Autodesk Fusion 360 part; units mm, degrees
(part 2 of 8)
  spline S57 degree 5 poles (-37.4182, -68.8904) (-37.4192, -68.8954) (-37.4245, -68.9203) (-37.434, -68.9652) (-37.4475, -69.03) (-37.4649, -69.1149) (-37.4849, -69.2149) (-37.5045, -69.315) (-37.5237, -69.4153) (-37.5425, -69.5158) (-37.5608, -69.6164) (-37.5788, -69.7172) (-37.5963, -69.8182) (-37.6135, -69.9192) (-37.6302, -70.0204) (-37.6466, -70.1218) (-37.6626, -70.2233) (-37.6782, -70.3249) (-37.6934, -70.4267) (-37.7082, -70.5286) (-37.7227, -70.6307) (-37.7368, -70.7328) (-37.7505, -70.8351) (-37.7639, -70.9376) (-37.7769, -71.0401) (-37.7895, -71.1428) (-37.8018, -71.2456) (-37.8137, -71.3485) (-37.8253, -71.4515) (-37.8365, -71.5546) (-37.8474, -71.6579) (-37.8579, -71.7612) (-37.8681, -71.8647) (-37.878, -71.9683) (-37.8875, -72.072) (-37.8966, -72.1758) (-37.9054, -72.2797) (-37.9139, -72.3837) (-37.9221, -72.4878) (-37.9283, -72.5712) (-37.9329, -72.6338) (-37.9358, -72.6755) (-37.9373, -72.6964) knots 0.467834 0.467834 0.467834 0.467834 0.467834 0.467834 0.471429 0.485714 0.5 0.514286 0.528571 0.542857 0.557143 0.571429 0.585714 0.6 0.614286 0.628571 0.642857 0.657143 0.671429 0.685714 0.7 0.714286 0.728571 0.742857 0.757143 0.771429 0.785714 0.8 0.814286 0.828571 0.842857 0.857143 0.871429 0.885714 0.9 0.914286 0.928571 0.942857 0.957143 0.971429 0.985714 1 1 1 1 1 1
  arc A29 (-37.9373, -72.6964) -> (-36.5136, -73.4218) centre (0, 0) ccw
  spline S58 degree 5 poles (-36.5136, -73.4218) (-36.4976, -73.4083) (-36.4656, -73.3814) (-36.4176, -73.3409) (-36.3538, -73.2869) (-36.2744, -73.2191) (-36.1952, -73.1511) (-36.1164, -73.0829) (-36.0378, -73.0144) (-35.9595, -72.9458) (-35.8815, -72.877) (-35.8037, -72.8079) (-35.7263, -72.7386) (-35.6491, -72.6692) (-35.5723, -72.5995) (-35.4958, -72.5295) (-35.4195, -72.4594) (-35.3436, -72.389) (-35.2679, -72.3185) (-35.1926, -72.2477) (-35.1176, -72.1767) (-35.0429, -72.1054) (-34.9686, -72.034) (-34.8945, -71.9623) (-34.8208, -71.8904) (-34.7474, -71.8183) (-34.6743, -71.7459) (-34.6016, -71.6733) (-34.5292, -71.6005) (-34.4572, -71.5274) (-34.3855, -71.4541) (-34.3142, -71.3806) (-34.2432, -71.3069) (-34.1726, -71.2329) (-34.1023, -71.1586) (-34.0324, -71.0842) (-33.9629, -71.0094) (-33.8938, -70.9345) (-33.8353, -70.8705) (-33.7908, -70.8215) (-33.7601, -70.7874) (-33.7431, -70.7685) (-33.7396, -70.7647) knots -1 -1 -1 -1 -1 -1 -0.985714 -0.971429 -0.957143 -0.942857 -0.928571 -0.914286 -0.9 -0.885714 -0.871429 -0.857143 -0.842857 -0.828571 -0.814286 -0.8 -0.785714 -0.771429 -0.757143 -0.742857 -0.728571 -0.714286 -0.7 -0.685714 -0.671429 -0.657143 -0.642857 -0.628571 -0.614286 -0.6 -0.585714 -0.571429 -0.557143 -0.542857 -0.528571 -0.514286 -0.5 -0.485714 -0.471429 -0.467834 -0.467834 -0.467834 -0.467834 -0.467834 -0.467834
  spline S59 degree 3 poles (-32.5768, -70.5256) (-32.695, -70.471) (-32.8228, -70.44) (-33.083, -70.4288) (-33.2129, -70.4486) (-33.4127, -70.5206) (-33.4862, -70.5579) (-33.6225, -70.6496) (-33.6847, -70.7036) (-33.7396, -70.7647) knots 0 0 0 0 0.039064 0.039064 0.078129 0.078129 0.102767 0.102767 0.127404 0.127404 0.127404 0.127404
  arc A30 (-32.5768, -70.5256) -> (-32.4711, -70.5744) centre (0, 0) ccw
  spline S60 degree 3 poles (-31.8977, -71.6138) (-31.8807, -71.4847) (-31.889, -71.3535) (-31.9555, -71.1017) (-32.013, -70.9835) (-32.141, -70.8142) (-32.1984, -70.755) (-32.3264, -70.6521) (-32.3965, -70.6087) (-32.4711, -70.5744) knots 0 0 0 0 0.039064 0.039064 0.078129 0.078129 0.102767 0.102767 0.127404 0.127404 0.127404 0.127404
  spline S61 degree 5 poles (-31.8977, -71.6138) (-31.8984, -71.6189) (-31.9018, -71.6442) (-31.9077, -71.6896) (-31.9161, -71.7553) (-31.9267, -71.8413) (-31.9389, -71.9425) (-31.9505, -72.0439) (-31.9618, -72.1454) (-31.9726, -72.2471) (-31.983, -72.3488) (-31.993, -72.4507) (-32.0026, -72.5527) (-32.0117, -72.6548) (-32.0205, -72.757) (-32.0289, -72.8594) (-32.0368, -72.9618) (-32.0444, -73.0644) (-32.0516, -73.167) (-32.0584, -73.2698) (-32.0648, -73.3726) (-32.0708, -73.4756) (-32.0765, -73.5786) (-32.0818, -73.6818) (-32.0867, -73.785) (-32.0912, -73.8884) (-32.0954, -73.9918) (-32.0992, -74.0953) (-32.1027, -74.199) (-32.1058, -74.3027) (-32.1085, -74.4065) (-32.1109, -74.5103) (-32.1129, -74.6143) (-32.1146, -74.7183) (-32.116, -74.8224) (-32.1169, -74.9266) (-32.1176, -75.0309) (-32.1179, -75.1353) (-32.1178, -75.2397) (-32.1175, -75.3233) (-32.1172, -75.386) (-32.1168, -75.4279) (-32.1167, -75.4488) knots 0.467834 0.467834 0.467834 0.467834 0.467834 0.467834 0.471429 0.485714 0.5 0.514286 0.528571 0.542857 0.557143 0.571429 0.585714 0.6 0.614286 0.628571 0.642857 0.657143 0.671429 0.685714 0.7 0.714286 0.728571 0.742857 0.757143 0.771429 0.785714 0.8 0.814286 0.828571 0.842857 0.857143 0.871429 0.885714 0.9 0.914286 0.928571 0.942857 0.957143 0.971429 0.985714 1 1 1 1 1 1
  arc A31 (-32.1167, -75.4488) -> (-30.6404, -76.0603) centre (0, 0) ccw
  spline S62 degree 5 poles (-30.6404, -76.0603) (-30.6255, -76.0456) (-30.5957, -76.0162) (-30.5511, -75.9721) (-30.4917, -75.9132) (-30.4179, -75.8394) (-30.3443, -75.7654) (-30.271, -75.6912) (-30.198, -75.6169) (-30.1254, -75.5423) (-30.053, -75.4675) (-29.9809, -75.3926) (-29.9091, -75.3175) (-29.8377, -75.2421) (-29.7666, -75.1666) (-29.6957, -75.0909) (-29.6252, -75.015) (-29.555, -74.9389) (-29.4852, -74.8626) (-29.4156, -74.7861) (-29.3464, -74.7095) (-29.2776, -74.6326) (-29.209, -74.5555) (-29.1408, -74.4783) (-29.073, -74.4008) (-29.0055, -74.3231) (-28.9383, -74.2452) (-28.8715, -74.1672) (-28.8051, -74.0889) (-28.739, -74.0104) (-28.6733, -73.9317) (-28.6079, -73.8528) (-28.543, -73.7737) (-28.4784, -73.6944) (-28.4141, -73.6149) (-28.3503, -73.5352) (-28.2869, -73.4552) (-28.2238, -73.3751) (-28.1706, -73.3067) (-28.1301, -73.2543) (-28.1021, -73.218) (-28.0866, -73.1978) (-28.0835, -73.1937) knots -1 -1 -1 -1 -1 -1 -0.985714 -0.971429 -0.957143 -0.942857 -0.928571 -0.914286 -0.9 -0.885714 -0.871429 -0.857143 -0.842857 -0.828571 -0.814286 -0.8 -0.785714 -0.771429 -0.757143 -0.742857 -0.728571 -0.714286 -0.7 -0.685714 -0.671429 -0.657143 -0.642857 -0.628571 -0.614286 -0.6 -0.585714 -0.571429 -0.557143 -0.542857 -0.528571 -0.514286 -0.5 -0.485714 -0.471429 -0.467834 -0.467834 -0.467834 -0.467834 -0.467834 -0.467834
  spline S63 degree 3 poles (-26.943, -72.8642) (-27.0652, -72.819) (-27.195, -72.7981) (-27.4552, -72.8073) (-27.5832, -72.8373) (-27.7767, -72.9248) (-27.8471, -72.9677) (-27.9757, -73.0698) (-28.0335, -73.1286) (-28.0835, -73.1937) knots 0 0 0 0 0.039064 0.039064 0.078129 0.078129 0.102767 0.102767 0.127404 0.127404 0.127404 0.127404
  arc A32 (-26.943, -72.8642) -> (-26.8339, -72.9045) centre (0, 0) ccw
  spline S64 degree 3 poles (-26.1807, -73.8957) (-26.1738, -73.7657) (-26.1924, -73.6356) (-26.2784, -73.3897) (-26.345, -73.2764) (-26.4859, -73.1176) (-26.5478, -73.0631) (-26.6835, -72.9706) (-26.7568, -72.9328) (-26.8339, -72.9045) knots 0 0 0 0 0.039064 0.039064 0.078129 0.078129 0.102767 0.102767 0.127404 0.127404 0.127404 0.127404
  spline S65 degree 5 poles (-26.1807, -73.8957) (-26.1809, -73.9008) (-26.1823, -73.9263) (-26.1846, -73.9721) (-26.1878, -74.0382) (-26.1917, -74.1248) (-26.1959, -74.2267) (-26.1995, -74.3286) (-26.2028, -74.4307) (-26.2056, -74.5329) (-26.208, -74.6352) (-26.2099, -74.7375) (-26.2115, -74.8399) (-26.2126, -74.9424) (-26.2133, -75.045) (-26.2136, -75.1477) (-26.2136, -75.2505) (-26.2131, -75.3533) (-26.2122, -75.4562) (-26.2109, -75.5592) (-26.2092, -75.6622) (-26.2072, -75.7653) (-26.2047, -75.8685) (-26.2019, -75.9718) (-26.1987, -76.0751) (-26.1951, -76.1785) (-26.1912, -76.2819) (-26.1868, -76.3854) (-26.1821, -76.489) (-26.1771, -76.5926) (-26.1717, -76.6963) (-26.1659, -76.8) (-26.1598, -76.9038) (-26.1533, -77.0077) (-26.1464, -77.1116) (-26.1393, -77.2155) (-26.1317, -77.3195) (-26.1238, -77.4236) (-26.1156, -77.5277) (-26.1087, -77.611) (-26.1034, -77.6735) (-26.0998, -77.7152) (-26.098, -77.736) knots 0.467834 0.467834 0.467834 0.467834 0.467834 0.467834 0.471429 0.485714 0.5 0.514286 0.528571 0.542857 0.557143 0.571429 0.585714 0.6 0.614286 0.628571 0.642857 0.657143 0.671429 0.685714 0.7 0.714286 0.728571 0.742857 0.757143 0.771429 0.785714 0.8 0.814286 0.828571 0.842857 0.857143 0.871429 0.885714 0.9 0.914286 0.928571 0.942857 0.957143 0.971429 0.985714 1 1 1 1 1 1
  arc A33 (-26.098, -77.736) -> (-24.5784, -78.2298) centre (0, 0) ccw
  spline S66 degree 5 poles (-24.5784, -78.2298) (-24.5646, -78.214) (-24.5372, -78.1824) (-24.4962, -78.135) (-24.4417, -78.0716) (-24.3738, -77.9922) (-24.3063, -77.9127) (-24.239, -77.8329) (-24.1721, -77.7531) (-24.1055, -77.673) (-24.0392, -77.5928) (-23.9733, -77.5125) (-23.9076, -77.4319) (-23.8423, -77.3512) (-23.7773, -77.2704) (-23.7126, -77.1893) (-23.6483, -77.1081) (-23.5843, -77.0268) (-23.5206, -76.9452) (-23.4573, -76.8635) (-23.3943, -76.7817) (-23.3317, -76.6996) (-23.2694, -76.6174) (-23.2075, -76.535) (-23.1459, -76.4525) (-23.0847, -76.3697) (-23.0239, -76.2868) (-22.9634, -76.2038) (-22.9033, -76.1205) (-22.8436, -76.0371) (-22.7843, -75.9535) (-22.7253, -75.8697) (-22.6667, -75.7858) (-22.6086, -75.7016) (-22.5508, -75.6173) (-22.4934, -75.5328) (-22.4364, -75.4482) (-22.3799, -75.3633) (-22.3322, -75.291) (-22.2959, -75.2356) (-22.2709, -75.1972) (-22.257, -75.1758) (-22.2542, -75.1715) knots -1 -1 -1 -1 -1 -1 -0.985714 -0.971429 -0.957143 -0.942857 -0.928571 -0.914286 -0.9 -0.885714 -0.871429 -0.857143 -0.842857 -0.828571 -0.814286 -0.8 -0.785714 -0.771429 -0.757143 -0.742857 -0.728571 -0.714286 -0.7 -0.685714 -0.671429 -0.657143 -0.642857 -0.628571 -0.614286 -0.6 -0.585714 -0.571429 -0.557143 -0.542857 -0.528571 -0.514286 -0.5 -0.485714 -0.471429 -0.467834 -0.467834 -0.467834 -0.467834 -0.467834 -0.467834
  spline S67 degree 3 poles (-21.1431, -74.7535) (-21.2684, -74.718) (-21.3994, -74.7074) (-21.6582, -74.737) (-21.7834, -74.7769) (-21.9695, -74.8793) (-22.0363, -74.9276) (-22.1565, -75.0395) (-22.2095, -75.1026) (-22.2542, -75.1715) knots 0 0 0 0 0.039064 0.039064 0.078129 0.078129 0.102767 0.102767 0.127404 0.127404 0.127404 0.127404
  arc A34 (-21.1431, -74.7535) -> (-21.0311, -74.7851) centre (0, 0) ccw
  spline S68 degree 3 poles (-20.3022, -75.722) (-20.3055, -75.5919) (-20.3342, -75.4636) (-20.4393, -75.2253) (-20.5146, -75.1175) (-20.6675, -74.9703) (-20.7335, -74.9208) (-20.876, -74.8392) (-20.9521, -74.8073) (-21.0311, -74.7851) knots 0 0 0 0 0.039064 0.039064 0.078129 0.078129 0.102767 0.102767 0.127404 0.127404 0.127404 0.127404
  spline S69 degree 5 poles (-20.3022, -75.722) (-20.302, -75.7272) (-20.3014, -75.7526) (-20.3001, -75.7985) (-20.2981, -75.8646) (-20.2952, -75.9512) (-20.2913, -76.0531) (-20.287, -76.1551) (-20.2822, -76.2571) (-20.277, -76.3592) (-20.2714, -76.4613) (-20.2653, -76.5635) (-20.2588, -76.6658) (-20.2519, -76.768) (-20.2446, -76.8704) (-20.2368, -76.9728) (-20.2287, -77.0752) (-20.2201, -77.1777) (-20.2111, -77.2802) (-20.2018, -77.3827) (-20.192, -77.4853) (-20.1819, -77.588) (-20.1714, -77.6906) (-20.1604, -77.7934) (-20.1491, -77.8961) (-20.1375, -77.9989) (-20.1254, -78.1017) (-20.113, -78.2045) (-20.1002, -78.3074) (-20.087, -78.4103) (-20.0735, -78.5133) (-20.0596, -78.6162) (-20.0453, -78.7192) (-20.0307, -78.8222) (-20.0157, -78.9253) (-20.0004, -79.0284) (-19.9847, -79.1314) (-19.9687, -79.2346) (-19.9523, -79.3377) (-19.939, -79.4202) (-19.9288, -79.4821) (-19.9219, -79.5234) (-19.9185, -79.544) knots 0.467834 0.467834 0.467834 0.467834 0.467834 0.467834 0.471429 0.485714 0.5 0.514286 0.528571 0.542857 0.557143 0.571429 0.585714 0.6 0.614286 0.628571 0.642857 0.657143 0.671429 0.685714 0.7 0.714286 0.728571 0.742857 0.757143 0.771429 0.785714 0.8 0.814286 0.828571 0.842857 0.857143 0.871429 0.885714 0.9 0.914286 0.928571 0.942857 0.957143 0.971429 0.985714 1 1 1 1 1 1
  arc A35 (-19.9185, -79.544) -> (-18.3648, -79.9171) centre (0, 0) ccw
  spline S70 degree 5 poles (-18.3648, -79.9171) (-18.3523, -79.9002) (-18.3275, -79.8666) (-18.2903, -79.816) (-18.2409, -79.7486) (-18.1795, -79.6641) (-18.1184, -79.5795) (-18.0576, -79.4948) (-17.9972, -79.4099) (-17.9371, -79.3249) (-17.8773, -79.2397) (-17.8178, -79.1544) (-17.7587, -79.069) (-17.6999, -78.9834) (-17.6414, -78.8977) (-17.5833, -78.8119) (-17.5256, -78.7259) (-17.4681, -78.6397) (-17.4111, -78.5534) (-17.3544, -78.467) (-17.298, -78.3805) (-17.242, -78.2938) (-17.1864, -78.2069) (-17.1311, -78.1199) (-17.0762, -78.0328) (-17.0217, -77.9455) (-16.9675, -77.8581) (-16.9138, -77.7706) (-16.8604, -77.6828) (-16.8074, -77.595) (-16.7548, -77.507) (-16.7026, -77.4189) (-16.6508, -77.3306) (-16.5994, -77.2421) (-16.5484, -77.1535) (-16.4978, -77.0648) (-16.4477, -76.9759) (-16.398, -76.8869) (-16.3561, -76.8111) (-16.3242, -76.753) (-16.3023, -76.7127) (-16.2902, -76.6903) (-16.2877, -76.6858) knots -1 -1 -1 -1 -1 -1 -0.985714 -0.971429 -0.957143 -0.942857 -0.928571 -0.914286 -0.9 -0.885714 -0.871429 -0.857143 -0.842857 -0.828571 -0.814286 -0.8 -0.785714 -0.771429 -0.757143 -0.742857 -0.728571 -0.714286 -0.7 -0.685714 -0.671429 -0.657143 -0.642857 -0.628571 -0.614286 -0.6 -0.585714 -0.571429 -0.557143 -0.542857 -0.528571 -0.514286 -0.5 -0.485714 -0.471429 -0.467834 -0.467834 -0.467834 -0.467834 -0.467834 -0.467834
  spline S71 degree 3 poles (-15.2129, -76.1819) (-15.3405, -76.1564) (-15.472, -76.1561) (-15.7276, -76.2059) (-15.8494, -76.2555) (-16.0268, -76.3722) (-16.0896, -76.4256) (-16.2007, -76.5465) (-16.2486, -76.6136) (-16.2877, -76.6858) knots 0 0 0 0 0.039064 0.039064 0.078129 0.078129 0.102767 0.102767 0.127404 0.127404 0.127404 0.127404
  arc A36 (-15.2129, -76.1819) -> (-15.0987, -76.2046) centre (0, 0) ccw
  spline S72 degree 3 poles (-14.2985, -77.0815) (-14.312, -76.952) (-14.3508, -76.8264) (-14.4742, -76.597) (-14.5577, -76.4955) (-14.7217, -76.3607) (-14.7914, -76.3166) (-14.9399, -76.2464) (-15.0182, -76.2206) (-15.0987, -76.2046) knots 0 0 0 0 0.039064 0.039064 0.078129 0.078129 0.102767 0.102767 0.127404 0.127404 0.127404 0.127404
  spline S73 degree 5 poles (-14.2985, -77.0815) (-14.298, -77.0866) (-14.2953, -77.1119) (-14.2905, -77.1575) (-14.2833, -77.2234) (-14.2736, -77.3095) (-14.2617, -77.4107) (-14.2494, -77.512) (-14.2367, -77.6134) (-14.2234, -77.7147) (-14.2098, -77.8161) (-14.1957, -77.9175) (-14.1812, -78.0189) (-14.1663, -78.1203) (-14.151, -78.2218) (-14.1352, -78.3232) (-14.1191, -78.4247) (-14.1025, -78.5262) (-14.0855, -78.6277) (-14.0681, -78.7292) (-14.0504, -78.8307) (-14.0322, -78.9322) (-14.0136, -79.0338) (-13.9947, -79.1353) (-13.9754, -79.2369) (-13.9557, -79.3384) (-13.9356, -79.44) (-13.9151, -79.5415) (-13.8943, -79.6431) (-13.8731, -79.7446) (-13.8515, -79.8462) (-13.8296, -79.9477) (-13.8073, -80.0493) (-13.7846, -80.1509) (-13.7616, -80.2524) (-13.7383, -80.354) (-13.7146, -80.4555) (-13.6905, -80.557) (-13.6661, -80.6586) (-13.6463, -80.7398) (-13.6312, -80.8007) (-13.6212, -80.8413) (-13.6161, -80.8616) knots 0.467834 0.467834 0.467834 0.467834 0.467834 0.467834 0.471429 0.485714 0.5 0.514286 0.528571 0.542857 0.557143 0.571429 0.585714 0.6 0.614286 0.628571 0.642857 0.657143 0.671429 0.685714 0.7 0.714286 0.728571 0.742857 0.757143 0.771429 0.785714 0.8 0.814286 0.828571 0.842857 0.857143 0.871429 0.885714 0.9 0.914286 0.928571 0.942857 0.957143 0.971429 0.985714 1 1 1 1 1 1
  arc A37 (-13.6161, -80.8616) -> (-12.0379, -81.1116) centre (0, 0) ccw
  spline S74 degree 5 poles (-12.0379, -81.1116) (-12.0268, -81.0938) (-12.0047, -81.0583) (-11.9716, -81.005) (-11.9277, -80.9339) (-11.8731, -80.8449) (-11.8188, -80.7558) (-11.7649, -80.6665) (-11.7113, -80.5772) (-11.658, -80.4877) (-11.6051, -80.3981) (-11.5525, -80.3084) (-11.5002, -80.2186) (-11.4483, -80.1287) (-11.3968, -80.0386) (-11.3456, -79.9485) (-11.2948, -79.8582) (-11.2443, -79.7678) (-11.1942, -79.6774) (-11.1444, -79.5867) (-11.095, -79.496) (-11.046, -79.4052) (-10.9973, -79.3143) (-10.9491, -79.2232) (-10.9012, -79.132) (-10.8537, -79.0408) (-10.8066, -78.9494) (-10.7598, -78.8579) (-10.7135, -78.7662) (-10.6675, -78.6745) (-10.622, -78.5826) (-10.5769, -78.4907) (-10.5322, -78.3986) (-10.4879, -78.3064) (-10.444, -78.2141) (-10.4005, -78.1217) (-10.3575, -78.0291) (-10.3149, -77.9364) (-10.2791, -77.8576) (-10.252, -77.7972) (-10.2333, -77.7553) (-10.2229, -77.732) (-10.2208, -77.7274) knots -1 -1 -1 -1 -1 -1 -0.985714 -0.971429 -0.957143 -0.942857 -0.928571 -0.914286 -0.9 -0.885714 -0.871429 -0.857143 -0.842857 -0.828571 -0.814286 -0.8 -0.785714 -0.771429 -0.757143 -0.742857 -0.728571 -0.714286 -0.7 -0.685714 -0.671429 -0.657143 -0.642857 -0.628571 -0.614286 -0.6 -0.585714 -0.571429 -0.557143 -0.542857 -0.528571 -0.514286 -0.5 -0.485714 -0.471429 -0.467834 -0.467834 -0.467834 -0.467834 -0.467834 -0.467834
  spline S75 degree 3 poles (-9.1888, -77.1407) (-9.3181, -77.1253) (-9.4492, -77.1353) (-9.7001, -77.2049) (-9.8176, -77.2639) (-9.9853, -77.3942) (-10.0437, -77.4524) (-10.145, -77.5817) (-10.1875, -77.6523) (-10.2208, -77.7274) knots 0 0 0 0 0.039064 0.039064 0.078129 0.078129 0.102767 0.102767 0.127404 0.127404 0.127404 0.127404
  arc A38 (-9.1888, -77.1407) -> (-9.0732, -77.1543) centre (0, 0) ccw
  spline S76 degree 3 poles (-8.2067, -77.9657) (-8.2303, -77.8377) (-8.2788, -77.7155) (-8.4198, -77.4965) (-8.511, -77.4019) (-8.6852, -77.2804) (-8.758, -77.2419) (-8.9116, -77.1835) (-8.9917, -77.1639) (-9.0732, -77.1543) knots 0 0 0 0 0.039064 0.039064 0.078129 0.078129 0.102767 0.102767 0.127404 0.127404 0.127404 0.127404
  spline S77 degree 5 poles (-8.2067, -77.9657) (-8.2057, -77.9708) (-8.2011, -77.9958) (-8.1927, -78.0409) (-8.1804, -78.106) (-8.164, -78.191) (-8.1442, -78.2911) (-8.124, -78.3911) (-8.1033, -78.4911) (-8.0822, -78.5911) (-8.0606, -78.6911) (-8.0386, -78.7911) (-8.0162, -78.8911) (-7.9934, -78.991) (-7.9701, -79.0909) (-7.9465, -79.1908) (-7.9224, -79.2907) (-7.8979, -79.3906) (-7.873, -79.4904) (-7.8477, -79.5903) (-7.8221, -79.6901) (-7.796, -79.7899) (-7.7695, -79.8896) (-7.7427, -79.9894) (-7.7154, -80.0891) (-7.6878, -80.1888) (-7.6598, -80.2884) (-7.6315, -80.3881) (-7.6027, -80.4877) (-7.5736, -80.5873) (-7.5442, -80.6868) (-7.5143, -80.7863) (-7.4841, -80.8858) (-7.4536, -80.9853) (-7.4227, -81.0847) (-7.3914, -81.1841) (-7.3598, -81.2835) (-7.3279, -81.3828) (-7.2955, -81.4822) (-7.2694, -81.5616) (-7.2497, -81.6211) (-7.2364, -81.6608) (-7.2298, -81.6807) knots 0.467834 0.467834 0.467834 0.467834 0.467834 0.467834 0.471429 0.485714 0.5 0.514286 0.528571 0.542857 0.557143 0.571429 0.585714 0.6 0.614286 0.628571 0.642857 0.657143 0.671429 0.685714 0.7 0.714286 0.728571 0.742857 0.757143 0.771429 0.785714 0.8 0.814286 0.828571 0.842857 0.857143 0.871429 0.885714 0.9 0.914286 0.928571 0.942857 0.957143 0.971429 0.985714 1 1 1 1 1 1
  arc A39 (-7.2298, -81.6807) -> (-5.6369, -81.806) centre (0, 0) ccw
  spline S78 degree 5 poles (-5.6369, -81.806) (-5.6272, -81.7875) (-5.6079, -81.7503) (-5.5791, -81.6946) (-5.5409, -81.6202) (-5.4934, -81.5272) (-5.4463, -81.4341) (-5.3996, -81.3409) (-5.3532, -81.2476) (-5.3071, -81.1542) (-5.2613, -81.0608) (-5.216, -80.9672) (-5.1709, -80.8736) (-5.1262, -80.7799) (-5.0819, -80.6861) (-5.038, -80.5922) (-4.9943, -80.4982) (-4.9511, -80.4042) (-4.9082, -80.31) (-4.8658, -80.2158) (-4.8236, -80.1215) (-4.7819, -80.0271) (-4.7405, -79.9326) (-4.6995, -79.838) (-4.6589, -79.7434) (-4.6187, -79.6487) (-4.5789, -79.5539) (-4.5395, -79.459) (-4.5005, -79.364) (-4.4619, -79.2689) (-4.4237, -79.1738) (-4.386, -79.0786) (-4.3486, -78.9833) (-4.3117, -78.8879) (-4.2752, -78.7924) (-4.2391, -78.6968) (-4.2035, -78.6012) (-4.1683, -78.5055) (-4.1388, -78.424) (-4.1165, -78.3617) (-4.1011, -78.3185) (-4.0926, -78.2945) (-4.0909, -78.2897) knots -1 -1 -1 -1 -1 -1 -0.985714 -0.971429 -0.957143 -0.942857 -0.928571 -0.914286 -0.9 -0.885714 -0.871429 -0.857143 -0.842857 -0.828571 -0.814286 -0.8 -0.785714 -0.771429 -0.757143 -0.742857 -0.728571 -0.714286 -0.7 -0.685714 -0.671429 -0.657143 -0.642857 -0.628571 -0.614286 -0.6 -0.585714 -0.571429 -0.557143 -0.542857 -0.528571 -0.514286 -0.5 -0.485714 -0.471429 -0.467834 -0.467834 -0.467834 -0.467834 -0.467834 -0.467834
  spline S79 degree 3 poles (-3.1081, -77.6238) (-3.2382, -77.6186) (-3.3681, -77.6388) (-3.6128, -77.728) (-3.7252, -77.796) (-3.8822, -77.939) (-3.9359, -78.0016) (-4.0267, -78.1385) (-4.0635, -78.2122) (-4.0909, -78.2897) knots 0 0 0 0 0.039064 0.039064 0.078129 0.078129 0.102767 0.102767 0.127404 0.127404 0.127404 0.127404
  arc A40 (-3.1081, -77.6238) -> (-2.9918, -77.6284) centre (0, 0) ccw
  spline S80 degree 3 poles (-2.0643, -78.3693) (-2.0979, -78.2435) (-2.1558, -78.1255) (-2.3135, -77.9183) (-2.4119, -77.8311) (-2.595, -77.7236) (-2.6707, -77.6909) (-2.8284, -77.6448) (-2.9097, -77.6315) (-2.9918, -77.6284) knots 0 0 0 0 0.039064 0.039064 0.078129 0.078129 0.102767 0.102767 0.127404 0.127404 0.127404 0.127404
  spline S81 degree 5 poles (-2.0643, -78.3693) (-2.0629, -78.3742) (-2.0563, -78.3988) (-2.0444, -78.4431) (-2.027, -78.507) (-2.004, -78.5905) (-1.9764, -78.6887) (-1.9484, -78.7868) (-1.92, -78.8849) (-1.8911, -78.983) (-1.8617, -79.081) (-1.832, -79.1789) (-1.8018, -79.2768) (-1.7712, -79.3746) (-1.7402, -79.4724) (-1.7087, -79.5702) (-1.6769, -79.6679) (-1.6447, -79.7655) (-1.612, -79.8631) (-1.579, -79.9607) (-1.5455, -80.0581) (-1.5117, -80.1556) (-1.4775, -80.2529) (-1.4429, -80.3503) (-1.4079, -80.4475) (-1.3726, -80.5448) (-1.3369, -80.6419) (-1.3008, -80.739) (-1.2643, -80.8361) (-1.2275, -80.9331) (-1.1903, -81.03) (-1.1527, -81.1269) (-1.1148, -81.2237) (-1.0766, -81.3205) (-1.038, -81.4172) (-0.999, -81.5138) (-0.9597, -81.6104) (-0.92, -81.7069) (-0.88, -81.8034) (-0.8478, -81.8805) (-0.8234, -81.9383) (-0.8071, -81.9768) (-0.7989, -81.9961) knots 0.467834 0.467834 0.467834 0.467834 0.467834 0.467834 0.471429 0.485714 0.5 0.514286 0.528571 0.542857 0.557143 0.571429 0.585714 0.6 0.614286 0.628571 0.642857 0.657143 0.671429 0.685714 0.7 0.714286 0.728571 0.742857 0.757143 0.771429 0.785714 0.8 0.814286 0.828571 0.842857 0.857143 0.871429 0.885714 0.9 0.914286 0.928571 0.942857 0.957143 0.971429 0.985714 1 1 1 1 1 1
  arc A41 (-0.7989, -81.9961) -> (0.7989, -81.9961) centre (0, 0) ccw
  spline S82 degree 5 poles (0.7989, -81.9961) (0.8071, -81.9768) (0.8234, -81.9383) (0.8478, -81.8805) (0.88, -81.8034) (0.92, -81.7069) (0.9597, -81.6104) (0.999, -81.5138) (1.038, -81.4172) (1.0766, -81.3205) (1.1148, -81.2237) (1.1527, -81.1269) (1.1903, -81.03) (1.2275, -80.9331) (1.2643, -80.8361) (1.3008, -80.739) (1.3369, -80.6419) (1.3726, -80.5448) (1.4079, -80.4475) (1.4429, -80.3503) (1.4775, -80.2529) (1.5117, -80.1556) (1.5455, -80.0581) (1.579, -79.9607) (1.612, -79.8631) (1.6447, -79.7655) (1.6769, -79.6679) (1.7087, -79.5702) (1.7402, -79.4724) (1.7712, -79.3746) (1.8018, -79.2768) (1.832, -79.1789) (1.8617, -79.081) (1.8911, -78.983) (1.92, -78.8849) (1.9484, -78.7868) (1.9764, -78.6887) (2.004, -78.5905) (2.027, -78.507) (2.0444, -78.4431) (2.0563, -78.3988) (2.0629, -78.3742) (2.0643, -78.3693) knots -1 -1 -1 -1 -1 -1 -0.985714 -0.971429 -0.957143 -0.942857 -0.928571 -0.914286 -0.9 -0.885714 -0.871429 -0.857143 -0.842857 -0.828571 -0.814286 -0.8 -0.785714 -0.771429 -0.757143 -0.742857 -0.728571 -0.714286 -0.7 -0.685714 -0.671429 -0.657143 -0.642857 -0.628571 -0.614286 -0.6 -0.585714 -0.571429 -0.557143 -0.542857 -0.528571 -0.514286 -0.5 -0.485714 -0.471429 -0.467834 -0.467834 -0.467834 -0.467834 -0.467834 -0.467834
  spline S83 degree 3 poles (2.9918, -77.6284) (2.8617, -77.6334) (2.7338, -77.6638) (2.4968, -77.7718) (2.3901, -77.8485) (2.2448, -78.0034) (2.1962, -78.07) (2.1164, -78.2135) (2.0855, -78.2899) (2.0643, -78.3693) knots 0 0 0 0 0.039064 0.039064 0.078129 0.078129 0.102767 0.102767 0.127404 0.127404 0.127404 0.127404
  arc A42 (2.9918, -77.6284) -> (3.1081, -77.6238) centre (0, 0) ccw
  spline S84 degree 3 poles (4.0909, -78.2897) (4.0475, -78.1669) (3.9805, -78.0538) (3.807, -77.8596) (3.7021, -77.7804) (3.5111, -77.6876) (3.4331, -77.661) (3.2723, -77.6274) (3.1901, -77.6205) (3.1081, -77.6238) knots 0 0 0 0 0.039064 0.039064 0.078129 0.078129 0.102767 0.102767 0.127404 0.127404 0.127404 0.127404
  spline S85 degree 5 poles (4.0909, -78.2897) (4.0926, -78.2945) (4.1011, -78.3185) (4.1165, -78.3617) (4.1388, -78.424) (4.1683, -78.5055) (4.2035, -78.6012) (4.2391, -78.6968) (4.2752, -78.7924) (4.3117, -78.8879) (4.3486, -78.9833) (4.386, -79.0786) (4.4237, -79.1738) (4.4619, -79.2689) (4.5005, -79.364) (4.5395, -79.459) (4.5789, -79.5539) (4.6187, -79.6487) (4.6589, -79.7434) (4.6995, -79.838) (4.7405, -79.9326) (4.7819, -80.0271) (4.8236, -80.1215) (4.8658, -80.2158) (4.9082, -80.31) (4.9511, -80.4042) (4.9943, -80.4982) (5.038, -80.5922) (5.0819, -80.6861) (5.1262, -80.7799) (5.1709, -80.8736) (5.216, -80.9672) (5.2613, -81.0608) (5.3071, -81.1542) (5.3532, -81.2476) (5.3996, -81.3409) (5.4463, -81.4341) (5.4934, -81.5272) (5.5409, -81.6202) (5.5791, -81.6946) (5.6079, -81.7503) (5.6272, -81.7875) (5.6369, -81.806) knots 0.467834 0.467834 0.467834 0.467834 0.467834 0.467834 0.471429 0.485714 0.5 0.514286 0.528571 0.542857 0.557143 0.571429 0.585714 0.6 0.614286 0.628571 0.642857 0.657143 0.671429 0.685714 0.7 0.714286 0.728571 0.742857 0.757143 0.771429 0.785714 0.8 0.814286 0.828571 0.842857 0.857143 0.871429 0.885714 0.9 0.914286 0.928571 0.942857 0.957143 0.971429 0.985714 1 1 1 1 1 1
  arc A43 (5.6369, -81.806) -> (7.2298, -81.6807) centre (0, 0) ccw
  spline S86 degree 5 poles (7.2298, -81.6807) (7.2364, -81.6608) (7.2497, -81.6211) (7.2694, -81.5616) (7.2955, -81.4822) (7.3279, -81.3828) (7.3598, -81.2835) (7.3914, -81.1841) (7.4227, -81.0847) (7.4536, -80.9853) (7.4841, -80.8858) (7.5143, -80.7863) (7.5442, -80.6868) (7.5736, -80.5873) (7.6027, -80.4877) (7.6315, -80.3881) (7.6598, -80.2884) (7.6878, -80.1888) (7.7154, -80.0891) (7.7427, -79.9894) (7.7695, -79.8896) (7.796, -79.7899) (7.8221, -79.6901) (7.8477, -79.5903) (7.873, -79.4904) (7.8979, -79.3906) (7.9224, -79.2907) (7.9465, -79.1908) (7.9701, -79.0909) (7.9934, -78.991) (8.0162, -78.8911) (8.0386, -78.7911) (8.0606, -78.6911) (8.0822, -78.5911) (8.1033, -78.4911) (8.124, -78.3911) (8.1442, -78.2911) (8.164, -78.191) (8.1804, -78.106) (8.1927, -78.0409) (8.2011, -77.9958) (8.2057, -77.9708) (8.2067, -77.9657) knots -1 -1 -1 -1 -1 -1 -0.985714 -0.971429 -0.957143 -0.942857 -0.928571 -0.914286 -0.9 -0.885714 -0.871429 -0.857143 -0.842857 -0.828571 -0.814286 -0.8 -0.785714 -0.771429 -0.757143 -0.742857 -0.728571 -0.714286 -0.7 -0.685714 -0.671429 -0.657143 -0.642857 -0.628571 -0.614286 -0.6 -0.585714 -0.571429 -0.557143 -0.542857 -0.528571 -0.514286 -0.5 -0.485714 -0.471429 -0.467834 -0.467834 -0.467834 -0.467834 -0.467834 -0.467834
  spline S87 degree 3 poles (9.0732, -77.1543) (8.9439, -77.1695) (8.8188, -77.2099) (8.591, -77.3362) (8.4906, -77.421) (8.3579, -77.5868) (8.3147, -77.657) (8.2464, -77.8064) (8.2216, -77.885) (8.2067, -77.9657) knots 0 0 0 0 0.039064 0.039064 0.078129 0.078129 0.102767 0.102767 0.127404 0.127404 0.127404 0.127404
  arc A44 (9.0732, -77.1543) -> (9.1888, -77.1407) centre (0, 0) ccw
  spline S88 degree 3 poles (10.2208, -77.7274) (10.1679, -77.6084) (10.0923, -77.5009) (9.904, -77.3209) (9.7933, -77.2501) (9.5956, -77.1726) (9.5157, -77.1522) (9.3528, -77.1313) (9.2703, -77.1309) (9.1888, -77.1407) knots 0 0 0 0 0.039064 0.039064 0.078129 0.078129 0.102767 0.102767 0.127404 0.127404 0.127404 0.127404
  spline S89 degree 5 poles (10.2208, -77.7274) (10.2229, -77.732) (10.2333, -77.7553) (10.252, -77.7972) (10.2791, -77.8576) (10.3149, -77.9364) (10.3575, -78.0291) (10.4005, -78.1217) (10.444, -78.2141) (10.4879, -78.3064) (10.5322, -78.3986) (10.5769, -78.4907) (10.622, -78.5826) (10.6675, -78.6745) (10.7135, -78.7662) (10.7598, -78.8579) (10.8066, -78.9494) (10.8537, -79.0408) (10.9012, -79.132) (10.9491, -79.2232) (10.9973, -79.3143) (11.046, -79.4052) (11.095, -79.496) (11.1444, -79.5867) (11.1942, -79.6774) (11.2443, -79.7678) (11.2948, -79.8582) (11.3456, -79.9485) (11.3968, -80.0386) (11.4483, -80.1287) (11.5002, -80.2186) (11.5525, -80.3084) (11.6051, -80.3981) (11.658, -80.4877) (11.7113, -80.5772) (11.7649, -80.6665) (11.8188, -80.7558) (11.8731, -80.8449) (11.9277, -80.9339) (11.9716, -81.005) (12.0047, -81.0583) (12.0268, -81.0938) (12.0379, -81.1116) knots 0.467834 0.467834 0.467834 0.467834 0.467834 0.467834 0.471429 0.485714 0.5 0.514286 0.528571 0.542857 0.557143 0.571429 0.585714 0.6 0.614286 0.628571 0.642857 0.657143 0.671429 0.685714 0.7 0.714286 0.728571 0.742857 0.757143 0.771429 0.785714 0.8 0.814286 0.828571 0.842857 0.857143 0.871429 0.885714 0.9 0.914286 0.928571 0.942857 0.957143 0.971429 0.985714 1 1 1 1 1 1
  arc A45 (12.0379, -81.1116) -> (13.6161, -80.8616) centre (0, 0) ccw
  spline S90 degree 5 poles (13.6161, -80.8616) (13.6212, -80.8413) (13.6312, -80.8007) (13.6463, -80.7398) (13.6661, -80.6586) (13.6905, -80.557) (13.7146, -80.4555) (13.7383, -80.354) (13.7616, -80.2524) (13.7846, -80.1509) (13.8073, -80.0493) (13.8296, -79.9477) (13.8515, -79.8462) (13.8731, -79.7446) (13.8943, -79.6431) (13.9151, -79.5415) (13.9356, -79.44) (13.9557, -79.3384) (13.9754, -79.2369) (13.9947, -79.1353) (14.0136, -79.0338) (14.0322, -78.9322) (14.0504, -78.8307) (14.0681, -78.7292) (14.0855, -78.6277) (14.1025, -78.5262) (14.1191, -78.4247) (14.1352, -78.3232) (14.151, -78.2218) (14.1663, -78.1203) (14.1812, -78.0189) (14.1957, -77.9175) (14.2098, -77.8161) (14.2234, -77.7147) (14.2367, -77.6134) (14.2494, -77.512) (14.2617, -77.4107) (14.2736, -77.3095) (14.2833, -77.2234) (14.2905, -77.1575) (14.2953, -77.1119) (14.298, -77.0866) (14.2985, -77.0815) knots -1 -1 -1 -1 -1 -1 -0.985714 -0.971429 -0.957143 -0.942857 -0.928571 -0.914286 -0.9 -0.885714 -0.871429 -0.857143 -0.842857 -0.828571 -0.814286 -0.8 -0.785714 -0.771429 -0.757143 -0.742857 -0.728571 -0.714286 -0.7 -0.685714 -0.671429 -0.657143 -0.642857 -0.628571 -0.614286 -0.6 -0.585714 -0.571429 -0.557143 -0.542857 -0.528571 -0.514286 -0.5 -0.485714 -0.471429 -0.467834 -0.467834 -0.467834 -0.467834 -0.467834 -0.467834
  spline S91 degree 3 poles (15.0987, -76.2046) (14.971, -76.2299) (14.8494, -76.2799) (14.6323, -76.4238) (14.5388, -76.5162) (14.4196, -76.6919) (14.382, -76.7652) (14.3256, -76.9195) (14.307, -76.9998) (14.2985, -77.0815) knots 0 0 0 0 0.039064 0.039064 0.078129 0.078129 0.102767 0.102767 0.127404 0.127404 0.127404 0.127404
  arc A46 (15.0987, -76.2046) -> (15.2129, -76.1819) centre (0, 0) ccw
  spline S92 degree 3 poles (16.2877, -76.6858) (16.2257, -76.5714) (16.1418, -76.4701) (15.94, -76.3055) (15.824, -76.2436) (15.6209, -76.1819) (15.5397, -76.1678) (15.3756, -76.1597) (15.2934, -76.1658) (15.2129, -76.1819) knots 0 0 0 0 0.039064 0.039064 0.078129 0.078129 0.102767 0.102767 0.127404 0.127404 0.127404 0.127404
  spline S93 degree 5 poles (16.2877, -76.6858) (16.2902, -76.6903) (16.3023, -76.7127) (16.3242, -76.753) (16.3561, -76.8111) (16.398, -76.8869) (16.4477, -76.9759) (16.4978, -77.0648) (16.5484, -77.1535) (16.5994, -77.2421) (16.6508, -77.3306) (16.7026, -77.4189) (16.7548, -77.507) (16.8074, -77.595) (16.8604, -77.6828) (16.9138, -77.7706) (16.9675, -77.8581) (17.0217, -77.9455) (17.0762, -78.0328) (17.1311, -78.1199) (17.1864, -78.2069) (17.242, -78.2938) (17.298, -78.3805) (17.3544, -78.467) (17.4111, -78.5534) (17.4681, -78.6397) (17.5256, -78.7259) (17.5833, -78.8119) (17.6414, -78.8977) (17.6999, -78.9834) (17.7587, -79.069) (17.8178, -79.1544) (17.8773, -79.2397) (17.9371, -79.3249) (17.9972, -79.4099) (18.0576, -79.4948) (18.1184, -79.5795) (18.1795, -79.6641) (18.2409, -79.7486) (18.2903, -79.816) (18.3275, -79.8666) (18.3523, -79.9002) (18.3648, -79.9171) knots 0.467834 0.467834 0.467834 0.467834 0.467834 0.467834 0.471429 0.485714 0.5 0.514286 0.528571 0.542857 0.557143 0.571429 0.585714 0.6 0.614286 0.628571 0.642857 0.657143 0.671429 0.685714 0.7 0.714286 0.728571 0.742857 0.757143 0.771429 0.785714 0.8 0.814286 0.828571 0.842857 0.857143 0.871429 0.885714 0.9 0.914286 0.928571 0.942857 0.957143 0.971429 0.985714 1 1 1 1 1 1
  arc A47 (18.3648, -79.9171) -> (19.9185, -79.544) centre (0, 0) ccw
  spline S94 degree 5 poles (19.9185, -79.544) (19.9219, -79.5234) (19.9288, -79.4821) (19.939, -79.4202) (19.9523, -79.3377) (19.9687, -79.2346) (19.9847, -79.1314) (20.0004, -79.0284) (20.0157, -78.9253) (20.0307, -78.8222) (20.0453, -78.7192) (20.0596, -78.6162) (20.0735, -78.5133) (20.087, -78.4103) (20.1002, -78.3074) (20.113, -78.2045) (20.1254, -78.1017) (20.1375, -77.9989) (20.1491, -77.8961) (20.1604, -77.7934) (20.1714, -77.6906) (20.1819, -77.588) (20.192, -77.4853) (20.2018, -77.3827) (20.2111, -77.2802) (20.2201, -77.1777) (20.2287, -77.0752) (20.2368, -76.9728) (20.2446, -76.8704) (20.2519, -76.768) (20.2588, -76.6658) (20.2653, -76.5635) (20.2714, -76.4613) (20.277, -76.3592) (20.2822, -76.2571) (20.287, -76.1551) (20.2913, -76.0531) (20.2952, -75.9512) (20.2981, -75.8646) (20.3001, -75.7985) (20.3014, -75.7526) (20.302, -75.7272) (20.3022, -75.722) knots -1 -1 -1 -1 -1 -1 -0.985714 -0.971429 -0.957143 -0.942857 -0.928571 -0.914286 -0.9 -0.885714 -0.871429 -0.857143 -0.842857 -0.828571 -0.814286 -0.8 -0.785714 -0.771429 -0.757143 -0.742857 -0.728571 -0.714286 -0.7 -0.685714 -0.671429 -0.657143 -0.642857 -0.628571 -0.614286 -0.6 -0.585714 -0.571429 -0.557143 -0.542857 -0.528571 -0.514286 -0.5 -0.485714 -0.471429 -0.467834 -0.467834 -0.467834 -0.467834 -0.467834 -0.467834
  spline S95 degree 3 poles (21.0311, -74.7851) (20.9058, -74.8203) (20.7885, -74.8797) (20.5833, -75.0401) (20.4974, -75.1396) (20.3923, -75.3241) (20.3606, -75.4002) (20.3165, -75.5584) (20.3043, -75.6399) (20.3022, -75.722) knots 0 0 0 0 0.039064 0.039064 0.078129 0.078129 0.102767 0.102767 0.127404 0.127404 0.127404 0.127404
  arc A48 (21.0311, -74.7851) -> (21.1431, -74.7535) centre (0, 0) ccw
  spline S96 degree 3 poles (22.2542, -75.1715) (22.1834, -75.0623) (22.0918, -74.9679) (21.8778, -74.8196) (21.7573, -74.767) (21.5499, -74.7214) (21.4678, -74.7137) (21.3036, -74.7186) (21.2221, -74.7311) (21.1431, -74.7535) knots 0 0 0 0 0.039064 0.039064 0.078129 0.078129 0.102767 0.102767 0.127404 0.127404 0.127404 0.127404
  spline S97 degree 5 poles (22.2542, -75.1715) (22.257, -75.1758) (22.2709, -75.1972) (22.2959, -75.2356) (22.3322, -75.291) (22.3799, -75.3633) (22.4364, -75.4482) (22.4934, -75.5328) (22.5508, -75.6173) (22.6086, -75.7016) (22.6667, -75.7858) (22.7253, -75.8697) (22.7843, -75.9535) (22.8436, -76.0371) (22.9033, -76.1205) (22.9634, -76.2038) (23.0239, -76.2868) (23.0847, -76.3697) (23.1459, -76.4525) (23.2075, -76.535) (23.2694, -76.6174) (23.3317, -76.6996) (23.3943, -76.7817) (23.4573, -76.8635) (23.5206, -76.9452) (23.5843, -77.0268) (23.6483, -77.1081) (23.7126, -77.1893) (23.7773, -77.2704) (23.8423, -77.3512) (23.9076, -77.4319) (23.9733, -77.5125) (24.0392, -77.5928) (24.1055, -77.673) (24.1721, -77.7531) (24.239, -77.8329) (24.3063, -77.9127) (24.3738, -77.9922) (24.4417, -78.0716) (24.4962, -78.135) (24.5372, -78.1824) (24.5646, -78.214) (24.5784, -78.2298) knots 0.467834 0.467834 0.467834 0.467834 0.467834 0.467834 0.471429 0.485714 0.5 0.514286 0.528571 0.542857 0.557143 0.571429 0.585714 0.6 0.614286 0.628571 0.642857 0.657143 0.671429 0.685714 0.7 0.714286 0.728571 0.742857 0.757143 0.771429 0.785714 0.8 0.814286 0.828571 0.842857 0.857143 0.871429 0.885714 0.9 0.914286 0.928571 0.942857 0.957143 0.971429 0.985714 1 1 1 1 1 1
  arc A49 (24.5784, -78.2298) -> (26.098, -77.736) centre (0, 0) ccw
  spline S98 degree 5 poles (26.098, -77.736) (26.0998, -77.7152) (26.1034, -77.6735) (26.1087, -77.611) (26.1156, -77.5277) (26.1238, -77.4236) (26.1317, -77.3195) (26.1393, -77.2155) (26.1464, -77.1116) (26.1533, -77.0077) (26.1598, -76.9038) (26.1659, -76.8) (26.1717, -76.6963) (26.1771, -76.5926) (26.1821, -76.489) (26.1868, -76.3854) (26.1912, -76.2819) (26.1951, -76.1785) (26.1987, -76.0751) (26.2019, -75.9718) (26.2047, -75.8685) (26.2072, -75.7653) (26.2092, -75.6622) (26.2109, -75.5592) (26.2122, -75.4562) (26.2131, -75.3533) (26.2136, -75.2505) (26.2136, -75.1477) (26.2133, -75.045) (26.2126, -74.9424) (26.2115, -74.8399) (26.2099, -74.7375) (26.208, -74.6352) (26.2056, -74.5329) (26.2028, -74.4307) (26.1995, -74.3286) (26.1959, -74.2267) (26.1917, -74.1248) (26.1878, -74.0382) (26.1846, -73.9721) (26.1823, -73.9263) (26.1809, -73.9008) (26.1807, -73.8957) knots -1 -1 -1 -1 -1 -1 -0.985714 -0.971429 -0.957143 -0.942857 -0.928571 -0.914286 -0.9 -0.885714 -0.871429 -0.857143 -0.842857 -0.828571 -0.814286 -0.8 -0.785714 -0.771429 -0.757143 -0.742857 -0.728571 -0.714286 -0.7 -0.685714 -0.671429 -0.657143 -0.642857 -0.628571 -0.614286 -0.6 -0.585714 -0.571429 -0.557143 -0.542857 -0.528571 -0.514286 -0.5 -0.485714 -0.471429 -0.467834 -0.467834 -0.467834 -0.467834 -0.467834 -0.467834
  spline S99 degree 3 poles (26.8339, -72.9045) (26.7117, -72.9494) (26.5994, -73.0178) (26.4075, -73.1939) (26.3296, -73.2998) (26.2393, -73.4919) (26.2136, -73.5703) (26.1821, -73.7315) (26.1763, -73.8137) (26.1807, -73.8957) knots 0 0 0 0 0.039064 0.039064 0.078129 0.078129 0.102767 0.102767 0.127404 0.127404 0.127404 0.127404
  arc A50 (26.8339, -72.9045) -> (26.943, -72.8642) centre (0, 0) ccw
  spline S100 degree 3 poles (28.0835, -73.1937) (28.0043, -73.0904) (27.9056, -73.0035) (27.6806, -72.8724) (27.5563, -72.8295) (27.346, -72.8003) (27.2636, -72.7991) (27.1003, -72.8168) (27.0201, -72.8357) (26.943, -72.8642) knots 0 0 0 0 0.039064 0.039064 0.078129 0.078129 0.102767 0.102767 0.127404 0.127404 0.127404 0.127404
  spline S101 degree 5 poles (28.0835, -73.1937) (28.0866, -73.1978) (28.1021, -73.218) (28.1301, -73.2543) (28.1706, -73.3067) (28.2238, -73.3751) (28.2869, -73.4552) (28.3503, -73.5352) (28.4141, -73.6149) (28.4784, -73.6944) (28.543, -73.7737) (28.6079, -73.8528) (28.6733, -73.9317) (28.739, -74.0104) (28.8051, -74.0889) (28.8715, -74.1672) (28.9383, -74.2452) (29.0055, -74.3231) (29.073, -74.4008) (29.1408, -74.4783) (29.209, -74.5555) (29.2776, -74.6326) (29.3464, -74.7095) (29.4156, -74.7861) (29.4852, -74.8626) (29.555, -74.9389) (29.6252, -75.015) (29.6957, -75.0909) (29.7666, -75.1666) (29.8377, -75.2421) (29.9091, -75.3175) (29.9809, -75.3926) (30.053, -75.4675) (30.1254, -75.5423) (30.198, -75.6169) (30.271, -75.6912) (30.3443, -75.7654) (30.4179, -75.8394) (30.4917, -75.9132) (30.5511, -75.9721) (30.5957, -76.0162) (30.6255, -76.0456) (30.6404, -76.0603) knots 0.467834 0.467834 0.467834 0.467834 0.467834 0.467834 0.471429 0.485714 0.5 0.514286 0.528571 0.542857 0.557143 0.571429 0.585714 0.6 0.614286 0.628571 0.642857 0.657143 0.671429 0.685714 0.7 0.714286 0.728571 0.742857 0.757143 0.771429 0.785714 0.8 0.814286 0.828571 0.842857 0.857143 0.871429 0.885714 0.9 0.914286 0.928571 0.942857 0.957143 0.971429 0.985714 1 1 1 1 1 1
  arc A51 (30.6404, -76.0603) -> (32.1167, -75.4488) centre (0, 0) ccw
  spline S102 degree 5 poles (32.1167, -75.4488) (32.1168, -75.4279) (32.1172, -75.386) (32.1175, -75.3233) (32.1178, -75.2397) (32.1179, -75.1353) (32.1176, -75.0309) (32.1169, -74.9266) (32.116, -74.8224) (32.1146, -74.7183) (32.1129, -74.6143) (32.1109, -74.5103) (32.1085, -74.4065) (32.1058, -74.3027) (32.1027, -74.199) (32.0992, -74.0953) (32.0954, -73.9918) (32.0912, -73.8884) (32.0867, -73.785) (32.0818, -73.6818) (32.0765, -73.5786) (32.0708, -73.4756) (32.0648, -73.3726) (32.0584, -73.2698) (32.0516, -73.167) (32.0444, -73.0644) (32.0368, -72.9618) (32.0289, -72.8594) (32.0205, -72.757) (32.0117, -72.6548) (32.0026, -72.5527) (31.993, -72.4507) (31.983, -72.3488) (31.9726, -72.2471) (31.9618, -72.1454) (31.9505, -72.0439) (31.9389, -71.9425) (31.9267, -71.8413) (31.9161, -71.7553) (31.9077, -71.6896) (31.9018, -71.6442) (31.8984, -71.6189) (31.8977, -71.6138) knots -1 -1 -1 -1 -1 -1 -0.985714 -0.971429 -0.957143 -0.942857 -0.928571 -0.914286 -0.9 -0.885714 -0.871429 -0.857143 -0.842857 -0.828571 -0.814286 -0.8 -0.785714 -0.771429 -0.757143 -0.742857 -0.728571 -0.714286 -0.7 -0.685714 -0.671429 -0.657143 -0.642857 -0.628571 -0.614286 -0.6 -0.585714 -0.571429 -0.557143 -0.542857 -0.528571 -0.514286 -0.5 -0.485714 -0.471429 -0.467834 -0.467834 -0.467834 -0.467834 -0.467834 -0.467834
  spline S103 degree 3 poles (32.4711, -70.5744) (32.3529, -70.6288) (32.2463, -70.7058) (32.0688, -70.8963) (31.9995, -71.008) (31.9245, -71.2067) (31.9051, -71.2868) (31.8863, -71.45) (31.887, -71.5324) (31.8977, -71.6138) knots 0 0 0 0 0.039064 0.039064 0.078129 0.078129 0.102767 0.102767 0.127404 0.127404 0.127404 0.127404
  arc A52 (32.4711, -70.5744) -> (32.5768, -70.5256) centre (0, 0) ccw
  spline S104 degree 3 poles (33.7396, -70.7647) (33.6526, -70.6679) (33.5474, -70.589) (33.3128, -70.476) (33.1855, -70.443) (32.9736, -70.4303) (32.8913, -70.4356) (32.7299, -70.4661) (32.6514, -70.4912) (32.5768, -70.5256) knots 0 0 0 0 0.039064 0.039064 0.078129 0.078129 0.102767 0.102767 0.127404 0.127404 0.127404 0.127404
  spline S105 degree 5 poles (33.7396, -70.7647) (33.7431, -70.7685) (33.7601, -70.7874) (33.7908, -70.8215) (33.8353, -70.8705) (33.8938, -70.9345) (33.9629, -71.0094) (34.0324, -71.0842) (34.1023, -71.1586) (34.1726, -71.2329) (34.2432, -71.3069) (34.3142, -71.3806) (34.3855, -71.4541) (34.4572, -71.5274) (34.5292, -71.6005) (34.6016, -71.6733) (34.6743, -71.7459) (34.7474, -71.8183) (34.8208, -71.8904) (34.8945, -71.9623) (34.9686, -72.034) (35.0429, -72.1054) (35.1176, -72.1767) (35.1926, -72.2477) (35.2679, -72.3185) (35.3436, -72.389) (35.4195, -72.4594) (35.4958, -72.5295) (35.5723, -72.5995) (35.6491, -72.6692) (35.7263, -72.7386) (35.8037, -72.8079) (35.8815, -72.877) (35.9595, -72.9458) (36.0378, -73.0144) (36.1164, -73.0829) (36.1952, -73.1511) (36.2744, -73.2191) (36.3538, -73.2869) (36.4176, -73.3409) (36.4656, -73.3814) (36.4976, -73.4083) (36.5136, -73.4218) knots 0.467834 0.467834 0.467834 0.467834 0.467834 0.467834 0.471429 0.485714 0.5 0.514286 0.528571 0.542857 0.557143 0.571429 0.585714 0.6 0.614286 0.628571 0.642857 0.657143 0.671429 0.685714 0.7 0.714286 0.728571 0.742857 0.757143 0.771429 0.785714 0.8 0.814286 0.828571 0.842857 0.857143 0.871429 0.885714 0.9 0.914286 0.928571 0.942857 0.957143 0.971429 0.985714 1 1 1 1 1 1
  arc A53 (36.5136, -73.4218) -> (37.9373, -72.6964) centre (0, 0) ccw
  spline S106 degree 5 poles (37.9373, -72.6964) (37.9358, -72.6755) (37.9329, -72.6338) (37.9283, -72.5712) (37.9221, -72.4878) (37.9139, -72.3837) (37.9054, -72.2797) (37.8966, -72.1758) (37.8875, -72.072) (37.878, -71.9683) (37.8681, -71.8647) (37.8579, -71.7612) (37.8474, -71.6579) (37.8365, -71.5546) (37.8253, -71.4515) (37.8137, -71.3485) (37.8018, -71.2456) (37.7895, -71.1428) (37.7769, -71.0401) (37.7639, -70.9376) (37.7505, -70.8351) (37.7368, -70.7328) (37.7227, -70.6307) (37.7082, -70.5286) (37.6934, -70.4267) (37.6782, -70.3249) (37.6626, -70.2233) (37.6466, -70.1218) (37.6302, -70.0204) (37.6135, -69.9192) (37.5963, -69.8182) (37.5788, -69.7172) (37.5608, -69.6164) (37.5425, -69.5158) (37.5237, -69.4153) (37.5045, -69.315) (37.4849, -69.2149) (37.4649, -69.1149) (37.4475, -69.03) (37.434, -68.9652) (37.4245, -68.9203) (37.4192, -68.8954) (37.4182, -68.8904) knots -1 -1 -1 -1 -1 -1 -0.985714 -0.971429 -0.957143 -0.942857 -0.928571 -0.914286 -0.9 -0.885714 -0.871429 -0.857143 -0.842857 -0.828571 -0.814286 -0.8 -0.785714 -0.771429 -0.757143 -0.742857 -0.728571 -0.714286 -0.7 -0.685714 -0.671429 -0.657143 -0.642857 -0.628571 -0.614286 -0.6 -0.585714 -0.571429 -0.557143 -0.542857 -0.528571 -0.514286 -0.5 -0.485714 -0.471429 -0.467834 -0.467834 -0.467834 -0.467834 -0.467834 -0.467834
  spline S107 degree 3 poles (37.9083, -67.8091) (37.7946, -67.8727) (37.6944, -67.9578) (37.5324, -68.1617) (37.472, -68.2785) (37.4129, -68.4824) (37.3998, -68.5638) (37.3939, -68.7279) (37.4011, -68.8101) (37.4182, -68.8904) knots 0 0 0 0 0.039064 0.039064 0.078129 0.078129 0.102767 0.102767 0.127404 0.127404 0.127404 0.127404
  arc A54 (37.9083, -67.8091) -> (38.0098, -67.7523) centre (0, 0) ccw
  spline S108 degree 3 poles (39.1878, -67.8994) (39.0934, -67.8097) (38.9823, -67.7393) (38.7396, -67.6451) (38.6101, -67.6221) (38.3978, -67.6262) (38.3162, -67.6378) (38.1577, -67.6809) (38.0814, -67.7121) (38.0098, -67.7523) knots 0 0 0 0 0.039064 0.039064 0.078129 0.078129 0.102767 0.102767 0.127404 0.127404 0.127404 0.127404
  spline S109 degree 5 poles (39.1878, -67.8994) (39.1915, -67.9029) (39.21, -67.9204) (39.2433, -67.9519) (39.2915, -67.9974) (39.3548, -68.0565) (39.4296, -68.1258) (39.5047, -68.1949) (39.5802, -68.2636) (39.6561, -68.3321) (39.7323, -68.4004) (39.8088, -68.4683) (39.8857, -68.536) (39.963, -68.6035) (40.0405, -68.6706) (40.1184, -68.7376) (40.1966, -68.8042) (40.2751, -68.8706) (40.3539, -68.9368) (40.433, -69.0027) (40.5125, -69.0683) (40.5922, -69.1337) (40.6723, -69.1989) (40.7526, -69.2638) (40.8333, -69.3285) (40.9142, -69.3929) (40.9954, -69.457) (41.0769, -69.521) (41.1587, -69.5847) (41.2408, -69.6481) (41.3232, -69.7114) (41.4058, -69.7743) (41.4887, -69.8371) (41.5719, -69.8996) (41.6553, -69.9619) (41.7391, -70.0239) (41.823, -70.0857) (41.9073, -70.1473) (41.9918, -70.2087) (42.0596, -70.2576) (42.1106, -70.2941) (42.1446, -70.3185) (42.1616, -70.3306) knots 0.467834 0.467834 0.467834 0.467834 0.467834 0.467834 0.471429 0.485714 0.5 0.514286 0.528571 0.542857 0.557143 0.571429 0.585714 0.6 0.614286 0.628571 0.642857 0.657143 0.671429 0.685714 0.7 0.714286 0.728571 0.742857 0.757143 0.771429 0.785714 0.8 0.814286 0.828571 0.842857 0.857143 0.871429 0.885714 0.9 0.914286 0.928571 0.942857 0.957143 0.971429 0.985714 1 1 1 1 1 1
  arc A55 (42.1616, -70.3306) -> (43.524, -69.4957) centre (0, 0) ccw
  spline S110 degree 5 poles (43.524, -69.4957) (43.521, -69.475) (43.5147, -69.4337) (43.5053, -69.3716) (43.4925, -69.289) (43.4762, -69.1859) (43.4596, -69.0829) (43.4426, -68.98) (43.4254, -68.8772) (43.4078, -68.7746) (43.3898, -68.6721) (43.3716, -68.5697) (43.353, -68.4675) (43.334, -68.3654) (43.3147, -68.2635) (43.2951, -68.1617) (43.2752, -68.06) (43.2548, -67.9585) (43.2342, -67.8572) (43.2132, -67.756) (43.1918, -67.6549) (43.1701, -67.554) (43.148, -67.4532) (43.1256, -67.3527) (43.1028, -67.2522) (43.0797, -67.152) (43.0561, -67.0519) (43.0322, -66.9519) (43.008, -66.8522) (42.9833, -66.7526) (42.9583, -66.6532) (42.9329, -66.5539) (42.9071, -66.4549) (42.8809, -66.356) (42.8543, -66.2573) (42.8273, -66.1588) (42.7999, -66.0605) (42.7721, -65.9624) (42.7481, -65.8791) (42.7296, -65.8155) (42.7166, -65.7716) (42.7094, -65.7471) (42.7079, -65.7422) knots -1 -1 -1 -1 -1 -1 -0.985714 -0.971429 -0.957143 -0.942857 -0.928571 -0.914286 -0.9 -0.885714 -0.871429 -0.857143 -0.842857 -0.828571 -0.814286 -0.8 -0.785714 -0.771429 -0.757143 -0.742857 -0.728571 -0.714286 -0.7 -0.685714 -0.671429 -0.657143 -0.642857 -0.628571 -0.614286 -0.6 -0.585714 -0.571429 -0.557143 -0.542857 -0.528571 -0.514286 -0.5 -0.485714 -0.471429 -0.467834 -0.467834 -0.467834 -0.467834 -0.467834 -0.467834
  spline S111 degree 3 poles (43.1116, -64.6259) (43.0033, -64.6981) (42.9101, -64.7908) (42.7646, -65.0068) (42.7136, -65.128) (42.6706, -65.3359) (42.664, -65.4181) (42.671, -65.5822) (42.6845, -65.6635) (42.7079, -65.7422) knots 0 0 0 0 0.039064 0.039064 0.078129 0.078129 0.102767 0.102767 0.127404 0.127404 0.127404 0.127404
  arc A56 (43.1116, -64.6259) -> (43.2084, -64.5612) centre (0, 0) ccw
  spline S112 degree 3 poles (44.3943, -64.6154) (44.2931, -64.5334) (44.1769, -64.472) (43.9275, -64.3971) (43.7967, -64.3843) (43.5853, -64.405) (43.5049, -64.4231) (43.3503, -64.4784) (43.2766, -64.5155) (43.2084, -64.5612) knots 0 0 0 0 0.039064 0.039064 0.078129 0.078129 0.102767 0.102767 0.127404 0.127404 0.127404 0.127404
  spline S113 degree 5 poles (44.3943, -64.6154) (44.3983, -64.6186) (44.4181, -64.6347) (44.4537, -64.6635) (44.5053, -64.705) (44.5731, -64.759) (44.6531, -64.8222) (44.7334, -64.8852) (44.8141, -64.9478) (44.8951, -65.0101) (44.9764, -65.0721) (45.0581, -65.1339) (45.1401, -65.1954) (45.2223, -65.2565) (45.3049, -65.3174) (45.3878, -65.378) (45.471, -65.4383) (45.5544, -65.4984) (45.6382, -65.5581) (45.7223, -65.6176) (45.8066, -65.6768) (45.8913, -65.7358) (45.9762, -65.7945) (46.0614, -65.8529) (46.1468, -65.911) (46.2326, -65.9689) (46.3186, -66.0265) (46.4049, -66.0838) (46.4914, -66.1409) (46.5782, -66.1977) (46.6653, -66.2543) (46.7526, -66.3106) (46.8402, -66.3666) (46.928, -66.4224) (47.0161, -66.478) (47.1044, -66.5333) (47.193, -66.5883) (47.2818, -66.6431) (47.3708, -66.6976) (47.4423, -66.741) (47.496, -66.7735) (47.5318, -66.7951) (47.5498, -66.8058) knots 0.467834 0.467834 0.467834 0.467834 0.467834 0.467834 0.471429 0.485714 0.5 0.514286 0.528571 0.542857 0.557143 0.571429 0.585714 0.6 0.614286 0.628571 0.642857 0.657143 0.671429 0.685714 0.7 0.714286 0.728571 0.742857 0.757143 0.771429 0.785714 0.8 0.814286 0.828571 0.842857 0.857143 0.871429 0.885714 0.9 0.914286 0.928571 0.942857 0.957143 0.971429 0.985714 1 1 1 1 1 1
  arc A57 (47.5498, -66.8058) -> (48.8425, -65.8666) centre (0, 0) ccw